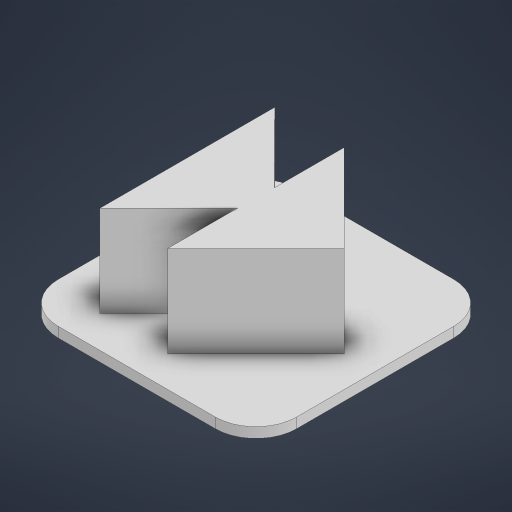
# Autodesk Inventor part: guzik_musik
Saved by Autodesk Inventor 2024.4 (Build 284460000, 460)
## iProperties
Created: 2026-03-18
Part Number: guzik_musik
Material: Ogólny
Document SubType Name: Modeling
Designer: User
Density: 1 g/cm^3
Appearance: Domyślna
Author: User
Autodesk Inventor part; units mm, degrees
ref_plane "YZ Plane" through (0, 0, 0) normal (1, 0, 0) x (0, 1, 0)
ref_plane "XZ Plane" through (0, 0, 0) normal (0, 1, 0) x (-1, 0, 0)
ref_plane "XY Plane" through (0, 0, 0) normal (0, 0, 1) x (1, 0, 0)
sketch "Szkic1" plane through (0, 0, 0) normal (0, 1, 0) x (-1, 0, 0)
  line L0 (4.0644, 4.4067) -> (-5.7356, 4.4067)
  line L1 (-5.7356, 4.4067) -> (-5.7356, -5.3933)
  line L2 (-5.7356, -5.3933) -> (4.0644, -5.3933)
  line L3 (4.0644, -5.3933) -> (4.0644, 4.4067)
  line L4 (4.0644, 4.4067) -> (-5.7356, -5.3933) construction
  line L5 (-5.7356, 4.4067) -> (4.0644, -5.3933) construction
  line L6 (-0.8356, -0.4933) -> (-0.8356, -4.9033)
  line L7 (-0.8356, -0.4933) -> (-5.2456, -0.4933)
  line L8 (-5.2456, -0.4933) -> (-0.8356, -4.9033)
  line L9 (-0.8356, -0.4933) -> (-1.796, -0.4933)
  line L10 (-0.8356, -0.4933) -> (2.5944, -0.4933)
  line L11 (-0.8356, -0.4933) -> (2.5944, -0.4933) construction
  line L12 (2.5944, -0.4933) -> (2.5944, -4.9033)
  line L13 (2.5944, -4.9033) -> (-1.796, -0.4933)
  line L14 (-5.2456, -0.4933) -> (-0.8356, 3.9167)
  line L15 (2.5944, 3.9167) -> (-1.796, -0.4933)
  line L16 (2.5944, -0.4933) -> (2.5944, 3.9167)
  line L17 (-0.8356, -0.4933) -> (-0.8356, 3.9167)
  line L18 (-6.7156, 5.3867) -> (5.0444, 5.3867)
  line L19 (5.0444, 5.3867) -> (5.0444, -6.3733)
  line L20 (5.0444, -6.3733) -> (-6.7156, -6.3733)
  line L21 (-6.7156, -6.3733) -> (-6.7156, 5.3867)
  line L22 (-6.7156, 5.3867) -> (5.0444, -6.3733) construction
  line L23 (5.0444, 5.3867) -> (-6.7156, -6.3733) construction
  point P0 (0, 0)
  point P1 (-0.8356, -1.458)
  point P2 (-0.8356, 0.4714)
  dimension "d0" = 9.8
  dimension "d1" = 9.8
  dimension "d2" = 4.41
  dimension "d3" = 4.41
  dimension "d4" = 0.9604
  dimension "d5" = 3.43
  dimension "d6" = 0
  dimension "d7" = 4.41
  dimension "d8" = 90
  dimension "d9" = 11.76
  dimension "d10" = 11.76
  constraints: 48 end point, 5 horizontal, 4 midpoint, 4 parallel, 3 perpendicular, 2 symmetric about line, 1 collinear, 1 point on line, 1 vertical
  measures "d0" distance of L3.start L2.start
  measures "d1" distance of L2.start L0.end
  measures "d2" distance of L10.start L6.end
  measures "d3" distance of L10.start L7.end
  measures "d4" distance of L10.start L9.end
  measures "d5" distance of L10.start L12.start
  measures "d6" distance between parallel lines of L10 L11
  measures "d7" distance of L12.start L12.end
  measures "d8" angle of L10 L12
  measures "d9" distance of L19.end L20.end
  measures "d10" distance of L18.end L19.end
extrude "Wyciągnięcie proste1" add sketch "Szkic1" along normal blind 0.5 contours L3 L2 L1 L0 | L10 L12 L13 L6 | L6 L13 L7 | L17 L15 L16 L10 | L7 L15 L17 | L6 L8 L7 L13 | L7 L14 L17 L15 | L18 L19 L20 L21
extrude "Wyciągnięcie proste2" add sketch "Szkic1" along normal blind 5 contours L10 L12 L13 L6 | L6 L13 L7 | L17 L15 L16 L10 | L7 L15 L17 | L6 L8 L7 L13 | L7 L14 L17 L15
fillet "Zaokrąglenie1" radius 2 4 edges at (6.7156, 0.25, 5.3867) (-5.0444, 0.25, 5.3867) (6.7156, 0.25, -6.3733) (-5.0444, 0.25, -6.3733)
offset faces "Rozmiar1" outward -0.04 faces at (2.3056, 2, 2.4467) (-1.4511, 2, 2.7682) (3.7756, 2, -1.9633) (0.8356, 2, -3.7549) (-0.3078, 2, -2.6064) (-2.5944, 3.5, -1.9633)
